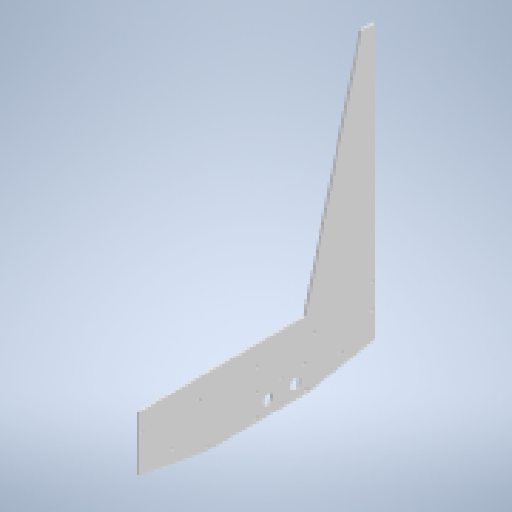
# Autodesk Inventor part: Outside Chassi Plate low 2.0
Saved by Autodesk Inventor 2023 (Build 270158000, 158)
## iProperties
Created: 2022-09-05
Part Number: Outside Chassi Plate low 2.0
Material: Generic
Document SubType Name: Modeling
Designer: deli
Density: 1 g/cm^3
Appearance: Default
Author: deli
Autodesk Inventor part; units mm, degrees
ref_plane "YZ Plane" through (0, 0, 0) normal (1, 0, 0) x (0, 1, 0)
ref_plane "XZ Plane" through (0, 0, 0) normal (0, 1, 0) x (-1, 0, 0)
ref_plane "XY Plane" through (0, 0, 0) normal (0, 0, 1) x (1, 0, 0)
sketch "Sketch1" plane through (0, 0, 0) normal (1, 0, 0) x (0, 1, 0)
  line L0 (-213.0456, 506.9498) -> (-293.8918, 506.9498)
  line L1 (-293.8918, 506.9498) -> (-312.9582, 406.3261)
  line L2 (-213.0456, 156.9498) -> (-293.8918, 156.9498)
  circle A0 centre (-285.0456, 456.9498) radius 2
  circle A1 centre (-285.0456, 456.9498) radius 48 construction
  arc A2 (-273.1215, 456.4048) -> (-296.9629, 457.629) centre (-285.0456, 456.9498) ccw construction
  circle A3 centre (-285.0456, 206.9498) radius 48 construction
  arc A4 (-296.901, 205.5596) -> (-273.1614, 208.0664) centre (-285.0456, 206.9498) ccw construction
  circle A5 centre (-285.0456, 206.9498) radius 2
  circle A6 centre (-292.2956, 315.7447) radius 7
  circle A7 centre (-292.2956, 275.607) radius 7
  circle A8 centre (-292.2956, 315.7447) radius 18.75 construction
  circle A9 centre (-292.2956, 275.607) radius 18.75 construction
  arc A10 (-305.0074, 316.4692) -> (-279.5765, 315.1634) centre (-292.2956, 315.7447) ccw construction
  arc A11 (-279.6191, 276.7981) -> (-304.9414, 274.1241) centre (-292.2956, 275.607) ccw construction
  line L3 (-273.1215, 456.4048) -> (-279.5765, 315.1634) construction
  line L4 (-305.0074, 316.4692) -> (-296.9629, 457.629) construction
  line L5 (-279.6191, 276.7981) -> (-273.1614, 208.0664) construction
  line L6 (-296.901, 205.5596) -> (-304.9414, 274.1241) construction
  circle A12 centre (-276.1617, 295.6759) radius 2
  circle A13 centre (-308.4296, 295.6759) radius 2
  circle A14 centre (-308.0456, 332.8474) radius 2
  circle A15 centre (-308.0456, 258.5044) radius 2
  circle A16 centre (-274.1266, 261.1002) radius 2
  circle A17 centre (-242.0456, 501.9498) radius 2
  arc A18 (-313.0456, 229.9036) -> (-313.0456, 229.9036) centre (-290.2956, 229.9036) ccw
  line L7 (-313.0456, 258.5044) -> (-313.0456, 229.9036)
  arc A19 (-312.9582, 406.3261) -> (-313.0456, 405.3952) centre (-308.0456, 405.3952) ccw
  line L8 (-313.0456, 405.3952) -> (-313.0456, 229.9036)
  line L9 (-293.8918, 156.9498) -> (-312.9582, 257.5735)
  circle A20 centre (-274.8437, 331.1068) radius 2
  arc A21 (-313.0456, 258.5044) -> (-312.9582, 257.5735) centre (-308.0456, 258.5044) ccw
  circle A22 centre (-242.0456, 246.9498) radius 2
  line L10 (-213.0456, 506.9498) -> (-213.0456, 302.8814)
  circle A23 centre (-242.0456, 416.9498) radius 2
  circle A24 centre (-242.0456, 331.9498) radius 2
  circle A25 centre (-308.0456, 405.3952) radius 2
  circle A26 centre (-242.0456, 161.9498) radius 2
  line L11 (-225.2933, 156.9498) -> (84.6394, 156.9498)
  line L12 (84.6394, 156.9498) -> (84.6394, 176.9498)
  line L13 (84.6394, 176.9498) -> (-213.0456, 302.8814)
  line L14 (-192.6416, 294.2497) -> (-200.4337, 275.8301)
  line L15 (-200.4337, 275.8301) -> (75.8605, 158.9476)
  line L16 (75.8605, 158.9476) -> (83.6526, 177.3672)
  circle A27 centre (-201.0456, 301.3338) radius 4.125
  circle A28 centre (130.5074, 161.0748) radius 4.125
  line L17 (56.8883, 166.9735) -> (56.1091, 165.1316)
  line L18 (56.1091, 165.1316) -> (75.4496, 156.9498)
  line L19 (75.4496, 156.9498) -> (76.2289, 158.7918)
  line L20 (76.2289, 158.7918) -> (75.8605, 158.9476)
  line L21 (75.8605, 158.9476) -> (75.0153, 156.9498)
  circle A29 centre (-182.7229, 279.1958) radius 1.5
  circle A30 centre (-58.3906, 226.5987) radius 1.5
  circle A31 centre (65.9418, 174.0015) radius 1.5
  point P0 (0, 0)
  point P1 (-199.9723, 297.3509)
  point P2 (-204.6514, 299.3303)
  dimension "d43" = 350
  dimension "d44" = 4
  dimension "d46" = 96
  dimension "d47" = 23.8732
  dimension "d48" = 96
  dimension "d49" = 4
  dimension "d51" = 23.8732
  dimension "d54" = 50
  dimension "d55" = 50
  dimension "d58" = 14
  dimension "d59" = 14
  dimension "d60" = 37.5
  dimension "d61" = 37.5
  dimension "d62" = 25.4648
  dimension "d63" = 25.4648
  dimension "d64" = 179.355
  dimension "d65" = 179.355
  dimension "d66" = 178.679
  dimension "d67" = 178.679
  dimension "d68" = 141.3888
  dimension "d70" = 69.0344
  dimension "d74" = 4
  dimension "d75" = 4
  dimension "d77" = 4
  dimension "d78" = 4
  dimension "d94" = 2.5
  dimension "d95" = 2.5
  dimension "d97" = 2.5
  dimension "d103" = 4
  dimension "d108" = 5
  dimension "d120" = 4
  dimension "d124" = 28
  dimension "d125" = 20.75
  dimension "d127" = 20.75
  dimension "d142" = 4
  dimension "d143" = 2.5
  dimension "d144" = 4
  dimension "d145" = 4
  dimension "d146" = 18
  dimension "d147" = 18
  dimension "d148" = 5
  dimension "d149" = 5
  dimension "d153" = 4
  dimension "d166" = 5
  dimension "d174" = 5
  dimension "d175" = 5
  dimension "d218" = 0
  dimension "d235" = 29
  dimension "d244" = 24
  dimension "d246" = 80.8462
  dimension "d247" = 80.8462
  dimension "d258" = 5
  dimension "d259" = 5
  dimension "d260" = 4
  dimension "d261" = 4
  dimension "d262" = 4
  dimension "d264" = 5
  dimension "d266" = 29
  dimension "d267" = 29
  dimension "d268" = 85
  dimension "d269" = 85
  dimension "d270" = 85
  dimension "d271" = 0
  dimension "d272" = 72.5479
  constraints: 44 end point, 32 centre point, 15 point on circle, 15 tangent, 8 perpendicular, 6 coincident, 6 point on line, 4 equal radius, 4 vertical, 3 concentric, 3 horizontal, 2 parallel, 1 collinear
  measures "d43" distance of L2.start L0.start
  measures "d44" diameter of A0
  measures "d46" diameter of A1
  measures "d47" diameter of A2
  measures "d48" diameter of A3
  measures "d49" diameter of A5
  measures "d51" diameter of A4
  measures "d54" distance from line of A0.centre L0
  measures "d55" distance from line of L2 A5.centre
  measures "d58" diameter of A6
  measures "d59" diameter of A7
  measures "d60" diameter of A8
  measures "d61" diameter of A9
  measures "d62" diameter of A10
  measures "d63" diameter of A11
  measures "d68" distance of L3.start L3.end
  measures "d70" distance of L5.start L5.end
  measures "d74" diameter of A14
  measures "d75" diameter of A13
  measures "d77" diameter of A12
  measures "d78" diameter of A16
  measures "d103" diameter of A17
  measures "d108" distance from line of L0 A17.centre
  measures "d120" diameter of A15
  measures "d124" distance from line of A0.centre L7
  measures "d125" distance from line of L7 A6.centre
  measures "d127" distance from line of L7 A7.centre
  measures "d142" distance from line of L5 A16.centre
  measures "d144" distance from line of L3 A20.centre
  measures "d145" diameter of A20
  measures "d146" distance from line of A0.centre L1
  measures "d147" distance from line of L9 A3.centre
  measures "d148" radius of A19
  measures "d149" radius of A21
  measures "d153" diameter of A22
  measures "d166" distance from line of L8 A14.centre
  measures "d218" horizontal distance of A0.centre A5.centre
  measures "d235" distance from line of L10 A17.centre
  measures "d244" distance edge to line of A1 L10
  measures "d246" distance of L2.start L2.end
  measures "d247" distance of L0.start L0.end
  measures "d260" diameter of A23
  measures "d261" diameter of A24
  measures "d262" diameter of A25
  measures "d264" distance from line of L8 A25.centre
  measures "d266" distance from line of L10 A23.centre
  measures "d267" distance from line of L10 A24.centre
  measures "d268" distance of A23.centre A17.centre
  measures "d269" distance of A24.centre A23.centre
  measures "d270" distance of A22.centre A24.centre
  measures "d271" distance of A25.centre A19.centre
  measures "d272" distance of A14.centre A25.centre
extrude "Extrusion1" add sketch "Sketch1" along normal blind 3.175 contours L10 L13 A27 L14 L15 L17 L18 L21 L11 L2 L9 A18 A5 A21 L8 A19 L1 L0 | L13 A27 | L13 L16 L15 L14 | A18 A5 L9 | L21 L18 L17 L15 picked at (-202.9159, 298.4232)
thread "Thread1" size "M3x0.5" class "6H" standard "ANSI Metric M Profile" full length
thread "Thread2" size "M3x0.5" class "6H" standard "ANSI Metric M Profile" full length
thread "Thread3" size "M3x0.5" class "6H" standard "ANSI Metric M Profile" full length
body "Solid1"
